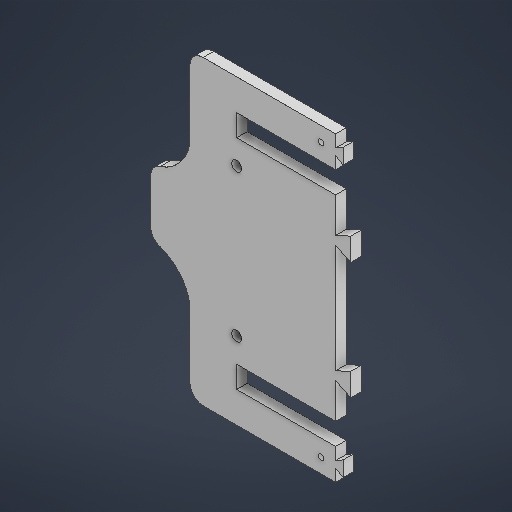
# Autodesk Inventor part: tmr
Saved by Autodesk Inventor 2026.1 (Build 301233020, 233B)
## iProperties
Created: 2026-01-27
Part Number: tmr
Material: Genérico
Document SubType Name: Sheet Metal
Designer: aylee
Density: 1 g/cm^3
Sheet Metal Rule: Por defecto_mm
Appearance: Valor por defecto
Author: aylee
Autodesk Inventor part; units mm, degrees
ref_plane "YZ Plane" through (0, 0, 0) normal (1, 0, 0) x (0, 1, 0)
ref_plane "XZ Plane" through (0, 0, 0) normal (0, 1, 0) x (-1, 0, 0)
ref_plane "XY Plane" through (0, 0, 0) normal (0, 0, 1) x (1, 0, 0)
sketch "Boceto1" plane through (0, 0, 0) normal (0, 0, 1) x (1, 0, 0)
  line L0 (0, 71.5) -> (84.4, 71.5)
  line L1 (0, 0) -> (4.5, 0)
  line L2 (62.2, 0) -> (62.2, 35)
  line L3 (62.2, 35) -> (112.2, 35)
  line L4 (112.2, 35) -> (112.2, 0)
  line L5 (84.4, 58.5) -> (84.4, 71.5)
  line L6 (84.4, 58.5) -> (0, 58.5)
  line L7 (87.2, 35) -> (108.2, 35)
  circle A0 centre (108.2, 46.75) radius 1.65
  circle A1 centre (66.2, 46.75) radius 1.65
  circle A2 centre (31.1, 43.75) radius 3
  circle A3 centre (178.7, 0) radius 2.5
  circle A4 centre (68.5, 81.35) radius 1.65
  line L8 (0, 90) -> (105.7, 90)
  arc A5 (120.7782, 83.1308) -> (105.7, 90) centre (105.672, 69.9553) ccw
  line L9 (200, 0) -> (200, 30.4)
  arc A6 (200, 30.4) -> (192, 38.4) centre (192, 30.4) ccw
  arc A7 (120.7782, 83.1308) -> (192, 38.4) centre (202.3119, 133.8853) ccw
  line L10 (4.5, 80.75) -> (4.5, 85.3)
  line L11 (4.5, 85.3) -> (0, 82.7)
  line L12 (4.5, 80.75) -> (4.5, 76.2)
  line L13 (4.5, 76.2) -> (0, 78.8)
  line L14 (0, 90) -> (0, 82.7)
  line L15 (0, 58.5) -> (0, 53.5)
  line L16 (0, 48.4) -> (0, 46.75)
  line L17 (0, 78.8) -> (0, 71.5)
  line L18 (0, 58.5) -> (0, 53.5)
  line L19 (0, 53.5) -> (0, 48.4)
  line L20 (0, 58.5) -> (0, 37.5)
  line L21 (9.1, 34.95) -> (9.1, 41.75)
  line L22 (9.1, 41.75) -> (0, 37.5)
  line L23 (9.1, 34.95) -> (9.1, 28.15)
  line L24 (9.1, 28.15) -> (0, 32.4)
  line L25 (0, 0) -> (0, 32.4)
  line L26 (0, 37.5) -> (0, 46.75)
  line L27 (0, -71.5) -> (84.4, -71.5)
  line L28 (62.2, 0) -> (62.2, -35)
  line L29 (62.2, -35) -> (112.2, -35)
  line L30 (112.2, -35) -> (112.2, 0)
  line L31 (84.4, -58.5) -> (84.4, -71.5)
  line L32 (84.4, -58.5) -> (0, -58.5)
  line L33 (87.2, -35) -> (108.2, -35)
  circle A8 centre (108.2, -46.75) radius 1.65
  circle A9 centre (66.2, -46.75) radius 1.65
  circle A10 centre (31.1, -43.75) radius 3
  circle A11 centre (178.7, 0) radius 2.5
  circle A12 centre (68.5, -81.35) radius 1.65
  line L34 (0, -90) -> (105.7, -90)
  arc A13 (105.7, -90) -> (120.7782, -83.1308) centre (105.672, -69.9553) ccw
  line L35 (200, 0) -> (200, -30.4)
  arc A14 (192, -38.4) -> (200, -30.4) centre (192, -30.4) ccw
  arc A15 (192, -38.4) -> (120.7782, -83.1308) centre (202.3119, -133.8853) ccw
  line L36 (4.5, -80.75) -> (4.5, -85.3)
  line L37 (4.5, -85.3) -> (0, -82.7)
  line L38 (4.5, -80.75) -> (4.5, -76.2)
  line L39 (4.5, -76.2) -> (0, -78.8)
  line L40 (0, -90) -> (0, -82.7)
  line L41 (0, -58.5) -> (0, -53.5)
  line L42 (0, -48.4) -> (0, -46.75)
  line L43 (0, -78.8) -> (0, -71.5)
  line L44 (0, -58.5) -> (0, -53.5)
  line L45 (0, -53.5) -> (0, -48.4)
  line L46 (0, -58.5) -> (0, -37.5)
  line L47 (9.1, -34.95) -> (9.1, -41.75)
  line L48 (9.1, -41.75) -> (0, -37.5)
  line L49 (9.1, -34.95) -> (9.1, -28.15)
  line L50 (9.1, -28.15) -> (0, -32.4)
  line L51 (0, 0) -> (0, -32.4)
  line L52 (0, -37.5) -> (0, -46.75)
  line L53 (261.8168, 58.5) -> (321.3628, 58.5)
  line L54 (321.3628, 58.5) -> (321.3628, -17.5)
  line L55 (321.3628, -17.5) -> (261.8168, -17.5)
  line L56 (261.8168, -17.5) -> (261.8168, 58.5)
  constraints: 114 end point, 33 symmetric about line, 16 centre point, 12 point on circle, 7 point on line, 5 vertical, 4 perpendicular, 2 parallel, 1 horizontal, 1 midpoint, 8 other
sketch "Boceto3" plane through (0, 0, 0) normal (0, 0, 1) x (1, 0, 0)
  line L0 (-258.9506, 92.2639) -> (-258.9506, 96.8139)
  line L1 (-258.9506, 96.8139) -> (-263.4506, 94.2139)
  line L2 (-258.9506, 92.2639) -> (-258.9506, 87.7139)
  line L3 (-258.9506, 87.7139) -> (-263.4506, 90.3139)
  line L4 (-263.4506, 101.5139) -> (-263.4506, 94.2139)
  line L5 (-263.4506, 70.0139) -> (-263.4506, 65.0139)
  line L6 (-263.4506, 59.9139) -> (-263.4506, 58.2639)
  line L7 (-263.4506, 90.3139) -> (-263.4506, 83.0139)
  line L8 (-263.4506, 70.0139) -> (-263.4506, 65.0139)
  line L9 (-263.4506, 65.0139) -> (-263.4506, 59.9139)
  line L10 (-263.4506, 70.0139) -> (-263.4506, 49.0139)
  line L11 (-254.3506, 46.4639) -> (-254.3506, 53.2639)
  line L12 (-254.3506, 53.2639) -> (-263.4506, 49.0139)
  line L13 (-254.3506, 46.4639) -> (-254.3506, 39.6639)
  line L14 (-254.3506, 39.6639) -> (-263.4506, 43.9139)
  line L15 (-263.4506, 11.5139) -> (-263.4506, 43.9139)
  line L16 (-263.4506, 49.0139) -> (-263.4506, 58.2639)
  line L17 (-263.4506, 83.0139) -> (-322.4506, 83.0139)
  line L18 (-263.4506, 83.0139) -> (-322.4506, 83.0139)
  line L19 (-263.4506, 70.0139) -> (-322.4506, 70.0139)
  line L20 (-322.4506, 70.0139) -> (-322.4506, 83.0139)
  circle A0 centre (-322.4506, 55.4139) radius 3
  line L21 (-350.4506, 83.0139) -> (-350.4506, 93.5139)
  circle A1 centre (-272.1006, 92.8639) radius 1.65
  line L22 (-342.4506, 101.5139) -> (-263.4506, 101.5139)
  line L23 (-373.8506, 11.5139) -> (-373.8506, 24.6339)
  arc A2 (-368.1081, 32.3088) -> (-373.8506, 24.6339) centre (-365.8506, 24.6339) ccw
  arc A3 (-342.4506, 101.5139) -> (-350.4506, 93.5139) centre (-342.4506, 93.5139) ccw
  arc A4 (-368.1081, 32.3088) -> (-350.4675, 52.85) centre (-376.4854, 57.3485) ccw
  line L24 (-350.4506, 83.0139) -> (-350.4506, 53.0604)
  arc A5 (-350.4675, 52.85) -> (-350.4506, 53.0604) centre (-357.2375, 53.5013) ccw
  line L25 (-258.9506, -69.2361) -> (-258.9506, -73.7861)
  line L26 (-258.9506, -73.7861) -> (-263.4506, -71.1861)
  line L27 (-258.9506, -69.2361) -> (-258.9506, -64.6861)
  line L28 (-258.9506, -64.6861) -> (-263.4506, -67.2861)
  line L29 (-263.4506, -78.4861) -> (-263.4506, -71.1861)
  line L30 (-263.4506, -46.9861) -> (-263.4506, -41.9861)
  line L31 (-263.4506, -36.8861) -> (-263.4506, -35.2361)
  line L32 (-263.4506, -67.2861) -> (-263.4506, -59.9861)
  line L33 (-263.4506, -46.9861) -> (-263.4506, -41.9861)
  line L34 (-263.4506, -41.9861) -> (-263.4506, -36.8861)
  line L35 (-263.4506, -46.9861) -> (-263.4506, -25.9861)
  line L36 (-254.3506, -23.4361) -> (-254.3506, -30.2361)
  line L37 (-254.3506, -30.2361) -> (-263.4506, -25.9861)
  line L38 (-254.3506, -23.4361) -> (-254.3506, -16.6361)
  line L39 (-254.3506, -16.6361) -> (-263.4506, -20.8861)
  line L40 (-263.4506, 11.5139) -> (-263.4506, -20.8861)
  line L41 (-263.4506, -25.9861) -> (-263.4506, -35.2361)
  line L42 (-263.4506, -59.9861) -> (-322.4506, -59.9861)
  line L43 (-263.4506, -59.9861) -> (-322.4506, -59.9861)
  line L44 (-263.4506, -46.9861) -> (-322.4506, -46.9861)
  line L45 (-322.4506, -46.9861) -> (-322.4506, -59.9861)
  circle A6 centre (-322.4506, -32.3861) radius 3
  line L46 (-350.4506, -59.9861) -> (-350.4506, -70.4861)
  circle A7 centre (-272.1006, -69.8361) radius 1.65
  line L47 (-342.4506, -78.4861) -> (-263.4506, -78.4861)
  line L48 (-373.8506, 11.5139) -> (-373.8506, -1.6061)
  arc A8 (-373.8506, -1.6061) -> (-368.1081, -9.2809) centre (-365.8506, -1.6061) ccw
  arc A9 (-350.4506, -70.4861) -> (-342.4506, -78.4861) centre (-342.4506, -70.4861) ccw
  arc A10 (-350.4675, -29.8221) -> (-368.1081, -9.2809) centre (-376.4854, -34.3207) ccw
  line L49 (-350.4506, -59.9861) -> (-350.4506, -30.0325)
  arc A11 (-350.4506, -30.0325) -> (-350.4675, -29.8221) centre (-357.2375, -30.4734) ccw
  point P0 (0, 0)
  constraints: 100 end point, 16 point on circle, 12 centre point, 6 point on line, 5 vertical, 2 horizontal, 2 tangent, 1 perpendicular
sketch "Boceto4" plane through (0, 0, 0) normal (0, 0, 1) x (1, 0, 0)
  line L0 (-279.0503, -82.5554) -> (-279.0503, -78.0054)
  line L1 (-279.0503, -78.0054) -> (-283.5503, -80.6054)
  line L2 (-279.0503, -82.5554) -> (-279.0503, -87.1054)
  line L3 (-279.0503, -87.1054) -> (-283.5503, -84.5054)
  line L4 (-283.5503, -73.3054) -> (-283.5503, -80.6054)
  line L5 (-283.5503, -104.8054) -> (-283.5503, -109.8054)
  line L6 (-283.5503, -114.9054) -> (-283.5503, -116.5554)
  line L7 (-283.5503, -84.5054) -> (-283.5503, -91.8054)
  line L8 (-283.5503, -104.8054) -> (-283.5503, -109.8054)
  line L9 (-283.5503, -109.8054) -> (-283.5503, -114.9054)
  line L10 (-283.5503, -104.8054) -> (-283.5503, -125.8054)
  line L11 (-274.4503, -128.3554) -> (-274.4503, -121.5554)
  line L12 (-274.4503, -121.5554) -> (-283.5503, -125.8054)
  line L13 (-274.4503, -128.3554) -> (-274.4503, -135.1554)
  line L14 (-274.4503, -135.1554) -> (-283.5503, -130.9054)
  line L15 (-283.5503, -163.3054) -> (-283.5503, -130.9054)
  line L16 (-283.5503, -125.8054) -> (-283.5503, -116.5554)
  line L17 (-393.9503, -163.3054) -> (-283.5503, -163.3054)
  line L18 (-283.5503, -91.8054) -> (-342.5503, -91.8054)
  line L19 (-283.5503, -91.8054) -> (-342.5503, -91.8054)
  line L20 (-283.5503, -104.8054) -> (-342.5503, -104.8054)
  line L21 (-342.5503, -104.8054) -> (-342.5503, -91.8054)
  circle A0 centre (-342.5503, -119.4054) radius 3
  line L22 (-370.5503, -91.8054) -> (-370.5503, -81.3054)
  circle A1 centre (-292.2003, -81.9554) radius 1.65
  line L23 (-362.5503, -73.3054) -> (-283.5503, -73.3054)
  line L24 (-393.9503, -163.3054) -> (-393.9503, -150.1854)
  arc A2 (-388.2078, -142.5105) -> (-393.9503, -150.1854) centre (-385.9503, -150.1854) ccw
  arc A3 (-362.5503, -73.3054) -> (-370.5503, -81.3054) centre (-362.5503, -81.3054) ccw
  arc A4 (-388.2078, -142.5105) -> (-370.5672, -121.9694) centre (-396.5851, -117.4708) ccw
  line L25 (-370.5503, -91.8054) -> (-370.5503, -121.7589)
  arc A5 (-370.5672, -121.9694) -> (-370.5503, -121.7589) centre (-377.3372, -121.318) ccw
  point P0 (0, 0)
  point P1 (89.2704, -12.3046)
  dimension "d61" = 13.12
  dimension "d62" = 8
  constraints: 52 end point, 8 point on circle, 6 centre point, 5 vertical, 3 point on line, 2 horizontal, 2 tangent, 1 perpendicular
  measures "d61" distance of L24.end L17.start
  measures "d62" radius of A3
extrude "Extrusión2" add sketch "Boceto3" along normal blind 6.35
fillet "Empalme3" radius 0.01 22 edges at (-348.1074, 99.1708, 6.35) (-350.4506, 88.2639, 6.35) (-302.9506, 101.5139, 6.35) (-356.4543, 40.1461, 6.35) (-373.8506, 18.0739, 6.35) (-372.256, -6.3988, 6.35) (-372.256, 29.4266, 6.35) (-356.4543, -17.1182, 6.35) (-348.1074, -76.1429, 6.35) (-302.9506, -78.4861, 6.35) (-350.4506, -45.0093, 6.35) (-348.1074, 99.1708, 0) (-350.4506, 88.2639, 0) (-302.9506, 101.5139, 0) (-356.4543, 40.1461, 0) (-373.8506, 18.0739, 0) (-372.256, -6.3988, 0) (-372.256, 29.4266, 0) (-356.4543, -17.1182, 0) (-348.1074, -76.1429, 0) (-302.9506, -78.4861, 0) (-350.4506, -45.0093, 0)
equation "\"Radio_pliegue\" = Grosor"
equation "\"Anchura_desahogo_plegado\" = Grosor"
equation "\"Profundidad_desahogo_plegado\" = 0.5 * Grosor"
equation "\"Tamaño_destalonado\" = 4 * Grosor"
equation "\"Remanente_mínimo\" = 2 * Grosor"
equation "\"Radiodetransición\" = Radio_pliegue"
equation "\"Tamaño_de_radio_de_Jacobi\" = Radio_pliegue"
equation "\"TamañoSeparación\" = Grosor"
equation "\"Grosor\" = 0.5"
